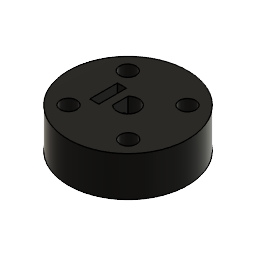
Wheel Hub v1 (Autodesk Fusion 360 design; units mm, degrees)
Autodesk Fusion 360 part; units mm, degrees
sketch "Sketch1" plane through (0, 0, 0) normal (0, 1, 0) x (1, 0, 0)
  circle A0 centre (0, 0) radius 12
  line L0 (-4.9, 2.78) -> (-4.9, -2.78)
  line L1 (-3.1, 2.78) -> (-4.9, 2.78)
  line L2 (-3.1, -2.78) -> (-3.1, 2.78)
  line L3 (-4.9, -2.78) -> (-3.1, -2.78)
  line L4 (0, 0) -> (5.3898, 0) construction
  line L5 (-1.5475, 1.5475) -> (-1.5475, -1.5475)
  arc A1 (-1.5475, -1.5475) -> (-1.5475, 1.5475) centre (0, 0) ccw
  line L6 (0, 0) -> (12, 0) construction
  line L7 (0, 0) -> (12, 0) construction
  circle A2 centre (-6.0104, 5.9604) radius 1.65
  line L8 (0, 0) -> (0, 12) construction
  line L9 (0, 0) -> (12, 0) construction
  line L10 (0, 0) -> (12, 0) construction
  circle A3 centre (6.0104, 5.9604) radius 1.65
  circle A4 centre (-6.0104, -5.9604) radius 1.65
  circle A5 centre (6.0104, -5.9604) radius 1.65
  line L11 (-6.0104, -9.1104) -> (-3.2824, -7.5354)
  line L12 (-3.2824, -7.5354) -> (-3.2824, -4.3854)
  line L13 (-3.2824, -4.3854) -> (-6.0104, -2.8104)
  line L14 (-6.0104, -2.8104) -> (-8.7384, -4.3854)
  line L15 (-8.7384, -4.3854) -> (-8.7384, -7.5354)
  line L16 (-8.7384, -7.5354) -> (-6.0104, -9.1104)
  line L17 (6.0104, -9.1104) -> (8.7384, -7.5354)
  line L18 (8.7384, -7.5354) -> (8.7384, -4.3854)
  line L19 (8.7384, -4.3854) -> (6.0104, -2.8104)
  line L20 (6.0104, -2.8104) -> (3.2824, -4.3854)
  line L21 (3.2824, -4.3854) -> (3.2824, -7.5354)
  line L22 (3.2824, -7.5354) -> (6.0104, -9.1104)
  line L23 (-6.0104, 2.8104) -> (-3.2824, 4.3854)
  line L24 (-3.2824, 4.3854) -> (-3.2824, 7.5354)
  line L25 (-3.2824, 7.5354) -> (-6.0104, 9.1104)
  line L26 (-6.0104, 9.1104) -> (-8.7384, 7.5354)
  line L27 (-8.7384, 7.5354) -> (-8.7384, 4.3854)
  line L28 (-8.7384, 4.3854) -> (-6.0104, 2.8104)
  line L29 (6.0104, 2.8104) -> (8.7384, 4.3854)
  line L30 (8.7384, 4.3854) -> (8.7384, 7.5354)
  line L31 (8.7384, 7.5354) -> (6.0104, 9.1104)
  line L32 (6.0104, 9.1104) -> (3.2824, 7.5354)
  line L33 (3.2824, 7.5354) -> (3.2824, 4.3854)
  line L34 (3.2824, 4.3854) -> (6.0104, 2.8104)
  point P0 (-6.0104, -5.9604)
  point P1 (6.0104, -5.9604)
  point P2 (-6.0104, 5.9604)
  point P3 (6.0104, 5.9604)
  dimension "d1" = 24
  dimension "d2" = 1.8
  dimension "d3" = 5.56
  dimension "d10" = 3.3
  dimension "d33" = 3.15
  dimension "d34" = 3.15
  dimension "d35" = 3.15
  dimension "d36" = 3.15
  constraint coincident A0.centre L4.start
  constraint horizontal L1
  constraint perpendicular L0 L1
  constraint parallel L1 L3
  constraint parallel L0 L2
  constraint concentric A0 A1
  constraint horizontal L4
  constraint vertical L5
  constraint horizontal L6
  constraint horizontal L7
  constraint coincident A0 L8.end
  constraint perpendicular L7 L8
  constraint symmetric A0.centre L6 L4.start
  constraint symmetric L7.end L6 L9.end
  constraint symmetric L6 A0.centre L4.start
  constraint symmetric L6 L7.end L9.end
  constraint symmetric A2 L8 A3
  constraint symmetric A2 L9 A4
  constraint symmetric L9 A3 A5
  constraint coincident P0 A4.centre
  constraint coincident P1 A5.centre
  constraint coincident P2 A2.centre
  constraint coincident P3 A3.centre
  measures "d1" diameter of A0
  measures "d2" distance of L2.start L0.end
  measures "d3" distance of L0.start L0.end
  measures "d10" diameter of A2
  measures "d33" distance of L11.start P0
  measures "d34" distance of L17.start P1
  measures "d35" distance of L23.start P2
  measures "d36" distance of L29.start P3
extrude "Extrude1" add sketch "Sketch1" along normal blind 8 contours A0 | L11 L12 L13 L14 L15 L16 | L17 L18 L19 L20 L21 L22 | L23 L24 L25 L26 L27 L28 | L29 L30 L31 L32 L33 L34
sketch "Sketch2" plane through (-1.5475, 0, 0) normal (1, 0, 0) x (0, 0, -1)
  line L0 (-1.5475, 0) -> (1.5475, 0)
  line L1 (1.5475, 0) -> (1.5475, 8)
  line L2 (1.5475, 8) -> (-1.5475, 8)
  line L3 (-1.5475, 8) -> (-1.5475, 0)
  line L4 (0, 8) -> (0, 0)
  line L5 (1.5475, 4) -> (-1.5475, 4)
  circle A0 centre (0, 4) radius 1.65
  dimension "d22" = 3.3
  constraint midpoint L2 L4.start
  constraint coincident L4.end origin
  constraint midpoint L1 L5.start
  constraint midpoint L3 L5.end
  constraint midpoint L5 A0.centre
  measures "d22" diameter of A0
extrude "Extrude2" cut sketch "Sketch2" against normal blind 13 contours L3 L4 L5 A0 | L1 L4 L5 A0 | L3 L4 L5 A0 | L1 L4 L5 A0
extrude "Extrude3" cut sketch "Sketch1" along normal blind 2 contours A3 | A5 | L11 L12 L13 L14 L15 L16 | L17 L18 L19 L20 L21 L22 | L23 L24 L25 L26 L27 L28 | L29 L30 L31 L32 L33 L34
ref_plane "WorkPlane1" through (-12.1, 4, 0) normal (-1, 0, 0) x (0, 0, 1)
sketch "Sketch3" plane through (-12.1, 0, 0) normal (-1, 0, 0) x (0, 0, 1)
  line L0 (0, 0) -> (0, 4)
  circle A0 centre (0, 4) radius 2.75
  dimension "d28" = 5.5
  constraint coincident L0.start origin
  constraint vertical L0
  constraint coincident L0.end A0.centre
  measures "d28" diameter of A0
extrude "Extrude4" cut sketch "Sketch3" against normal blind 2.2
extrude "Extrude5" add sketch "Sketch1" along normal blind 1.5 contours L0 L1 L2 L3
